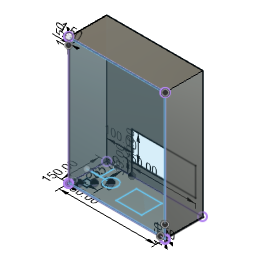
camera_box (Autodesk Fusion 360 design; units mm, degrees)
Autodesk Fusion 360 part; units mm, degrees
sketch "スケッチ1" plane through (0, 0, 0) normal (0, 1, 0) x (1, 0, 0)
  line L0 (0, 0) -> (380, 0)
  line L1 (380, 0) -> (380, 150)
  line L2 (380, 150) -> (0, 150)
  line L3 (0, 150) -> (0, 0)
  dimension "d1" = 380
  dimension "d2" = 150
  constraint horizontal L0
  constraint vertical L1
  constraint horizontal L2
  constraint vertical L3
  constraint coincident L0.start L3.end
  measures "d1" distance of L0.start L0.end
  measures "d2" distance of L0.start L2.end
extrude "押し出し1" add sketch "スケッチ1" along normal blind 500
sketch "スケッチ2" plane through (0, 0, 0) normal (0, 0, 1) x (1, 0, 0)
  line L0 (0, 0) -> (380, 0)
  line L1 (380, 0) -> (380, 500)
  line L2 (380, 500) -> (0, 500)
  line L3 (0, 500) -> (0, 0)
sketch "スケッチ3" plane through (0, 0, 0) normal (0, 0, 1) x (1, 0, 0)
  line L0 (380, 500) -> (0, 500)
  line L1 (380.7982, 500) -> (380.7982, 498.5)
  line L2 (0, 500) -> (0, 0)
  line L3 (0, 471) -> (1.5, 471)
  line L4 (1.5, 471) -> (1.5, 502)
  line L5 (380, 0) -> (380, 500)
  line L6 (380, 50) -> (378.5, 50)
  line L7 (378.5, 50) -> (377, 50)
  line L8 (0, 0) -> (380, 0)
  line L9 (361, 0) -> (361, 1.5)
  line L10 (378.5, 1.5) -> (1.5, 1.5)
  line L11 (1.5, 1.5) -> (1.5, 498.5115)
  line L12 (1.5, 498.5115) -> (378.5, 498.5115)
  line L13 (378.5, 498.5115) -> (378.5, 1.5)
  dimension "d5" = 1.5
  dimension "d6" = 1.5
  dimension "d7" = 1.5
  dimension "d10" = 1.5
  constraint coincident L0 L1.start
  constraint vertical L1
  constraint coincident L2 L3.start
  constraint perpendicular L2 L3
  constraint perpendicular L0 L4
  constraint coincident L5 L6.start
  constraint perpendicular L5 L6
  constraint horizontal L7
  constraint coincident L8 L9.start
  constraint perpendicular L8 L9
  constraint horizontal L10
  constraint vertical L11
  constraint horizontal L12
  constraint vertical L13
  constraint coincident L4 L11.end
  measures "d5" distance of L1.start L1.end
  measures "d6" distance of L3.start L3.end
  measures "d7" distance of L6.start L6.end
  measures "d10" distance of L9.start L9.end
extrude "押し出し2" cut sketch "スケッチ3" against normal blind 148.5 contours L4 L10 L11 L12 L13
sketch "スケッチ4" plane through (0, 0, -150) normal (0, 0, -1) x (-1, 0, 0)
  line L0 (-380, 0) -> (0, 0)
  line L1 (0, 0) -> (0, 500)
  line L2 (0, 500) -> (-380, 500)
  line L3 (-380, 500) -> (-380, 0)
  line L4 (0, 0) -> (-100, 0)
  line L5 (-100, 0) -> (-100, 50)
  line L6 (-100, 50) -> (-350, 50)
  line L7 (-350, 50) -> (-350, 160)
  line L8 (-350, 160) -> (-100, 160)
  line L9 (-100, 160) -> (-100, 50)
  dimension "d13" = 100
  dimension "d14" = 50
  dimension "d15" = 250
  dimension "d16" = 110
  constraint coincident L0.end L1.start
  constraint coincident L0 L4.end
  constraint perpendicular L4 L5
  constraint horizontal L6
  constraint vertical L7
  constraint horizontal L8
  constraint vertical L9
  measures "d13" distance of L0.end L4.end
  measures "d14" distance of L4.end L5.end
  measures "d15" distance of L5.end L6.end
  measures "d16" distance of L5.end L8.end
extrude "押し出し3" cut sketch "スケッチ4" against normal blind 30 contours L6 L7 L8 L9
sketch "スケッチ5" plane through (0, 0, 0) normal (0, 0, 1) x (1, 0, 0)
  line L0 (378.5, 1.5, -148.5) -> (1.5, 1.5, -148.5)
  line L1 (41.5712, 1.5, -148.5) -> (41.5712, 1.5, -83.5)
  line L2 (41.5712, 1.5, -83.5) -> (-11.7614, 1.5, -83.5)
  line L3 (1.5, 1.5, -83.5) -> (83.5, 1.5, -83.5)
  circle A0 through (87.5, 1.5, -83.5) (81.5, 1.5, -80.0359) (81.5, 1.5, -86.9641)
  dimension "d19" = 65
  dimension "d24" = 82
sketch "スケッチ6" plane through (0, 0, 0) normal (0, 0, 1) x (1, 0, 0)
sketch "スケッチ7" plane through (0, 0, 0) normal (0, 1, 0) x (1, 0, 0)
sketch "スケッチ8" plane through (0, 0, 0) normal (0, 0, 1) x (1, 0, 0)
  line L0 (1.5, 1.5, 0) -> (1.5, 1.5, -148.5)
  line L1 (1.5, 1.5, -18.4401) -> (21.5, 1.5, -18.4401)
  line L2 (378.5, 1.5) -> (1.5, 1.5)
  line L3 (21.5, 1.5, -18.4401) -> (21.5, 1.5, 0)
  line L4 (21.5, 1.5, -20) -> (51.5, 1.5, -20)
  line L5 (51.5, 1.5, -20) -> (51.5, 1.5, -50)
  line L6 (51.5, 1.5, -50) -> (21.5, 1.5, -50)
  line L7 (21.5, 1.5, -50) -> (21.5, 1.5, -20)
  circle A0 through (108.5, 1.5, -83.5) (71, 1.5, -61.8494) (71, 1.5, -105.1506)
  point P0 (83.5, 1.5)
  dimension "d26" = 20
  dimension "d27" = 20
  dimension "d28" = 30
  dimension "d29" = 30
  dimension "d30" = 50
sketch "スケッチ9" plane through (0, 0, 0) normal (0, 0, 1) x (1, 0, 0)
  line L0 (21.5, 1.5, -20) -> (51.5, 1.5, -20)
  line L1 (51.5, 1.5, -20) -> (51.5, 1.5, -50)
  line L2 (51.5, 1.5, -50) -> (21.5, 1.5, -50)
  line L3 (21.5, 1.5, -50) -> (21.5, 1.5, -20)
  point P0 (21.5, 1.5)
  point P1 (51.5, 1.5)
sketch "スケッチ10" plane through (0, 0, 0) normal (0, 0, 1) x (1, 0, 0)
  line L0 (153.9573, 1.5, -113.4079) -> (253.9573, 1.5, -113.4079)
  line L1 (253.9573, 1.5, -113.4079) -> (253.9573, 1.5, -33.4079)
  line L2 (253.9573, 1.5, -33.4079) -> (153.9573, 1.5, -33.4079)
  line L3 (153.9573, 1.5, -33.4079) -> (153.9573, 1.5, -113.4079)
  dimension "d31" = 100
  dimension "d32" = 80
